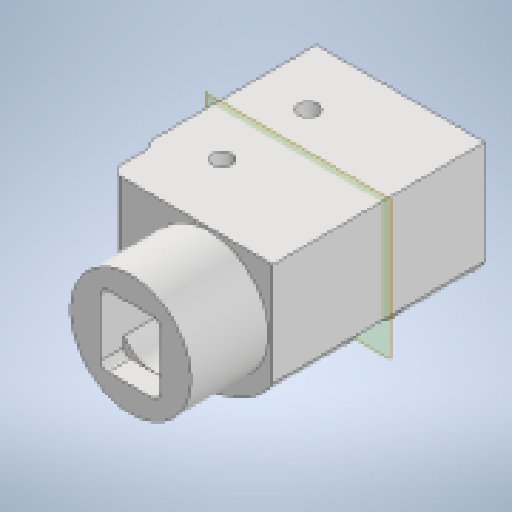
# Autodesk Inventor part: mototrs_Mount_miras_pololu_n20
Saved by Autodesk Inventor 2023.5 (Build 275446000, 446)
## iProperties
Created: 2025-04-06
Part Number: mototrs_Mount_miras_pololu_n20
Material: Ogólny
Document SubType Name: Modeling
Designer: kamil
Density: 1 g/cm^3
Appearance: Domyślna
Author: kamil
Autodesk Inventor part; units mm, degrees
ref_plane "YZ Plane" through (0, 0, 0) normal (1, 0, 0) x (0, 1, 0)
ref_plane "XZ Plane" through (0, 0, 0) normal (0, 1, 0) x (-1, 0, 0)
ref_plane "XY Plane" through (0, 0, 0) normal (0, 0, 1) x (1, 0, 0)
sketch "Szkic1" plane through (0, 0, 0) normal (0, 1, 0) x (-1, 0, 0)
  line L0 (22.5813, 6.7031) -> (-6.8457, 6.7031)
  line L1 (-6.8457, 6.7031) -> (-6.8457, -29.2969)
  line L2 (-6.8457, -29.2969) -> (22.5813, -29.2969)
  line L3 (22.5813, -29.2969) -> (22.5813, 6.7031)
  point P0 (0, 0)
  dimension "d0" = 36
  dimension "d1" = 29.427
  constraints: 8 end point, 2 parallel, 1 horizontal, 1 perpendicular
  measures "d0" distance of L1.end L0.end
  measures "d1" distance of L0.start L0.end
extrude "Wyciągnięcie proste1" add sketch "Szkic1" along normal blind 22
sketch "Szkic2" plane through (-22.5813, 0, 6.7031) normal (0, 0, 1) x (1, 0, 0)
  arc A0 (23.1002, 14.25) -> (13.1002, 14.2503) centre (18.1001, 11.0797) ccw projected
  arc A1 (13.1002, 7.75) -> (23.1002, 7.7503) centre (18.1001, 10.9206) ccw projected
  line L0 (23.1002, 7.7503) -> (23.1002, 14.25)
  line L1 (13.1002, 14.2503) -> (13.1002, 7.75)
  arc A2 (23.2002, 14.2789) -> (13.0002, 14.2792) centre (18.1001, 11.0797) ccw
  line L2 (23.2002, 14.2789) -> (23.2002, 7.7214)
  arc A3 (13.0002, 7.7211) -> (23.2002, 7.7214) centre (18.1001, 10.9206) ccw
  line L3 (13.0002, 7.7211) -> (13.0002, 14.2792)
  point P0 (22.5813, 0)
  dimension "d4" = 0.1
  constraints: 8 end point, 4 point on circle, 2 centre point, 2 parallel, 1 vertical, 3 other
  measures "d4" radial gap between concentric circles of A0 A2
extrude "Wyciągnięcie proste2" cut sketch "Szkic2" against normal blind 5 contours L0 A1 L1 A0 | L2 A3 L3 A2
sketch "Szkic3" plane through (-22.5813, 0, 1.7031) normal (0, 0, 1) x (1, 0, 0)
  line L0 (23.2002, 14.2789) -> (23.2002, 7.7214) projected
  arc A0 (23.2002, 14.2789) -> (13.0002, 14.2792) centre (18.1001, 11.0797) ccw projected
  line L1 (13.0002, 7.7211) -> (13.0002, 14.2792) projected
  arc A1 (13.0002, 7.7211) -> (23.2002, 7.7214) centre (18.1001, 10.9206) ccw projected
  arc A2 (21.7002, 13.8135) -> (14.5002, 13.8137) centre (18.1001, 11.0797) ccw
  line L2 (21.7002, 13.8135) -> (21.7002, 8.1867)
  arc A3 (14.5002, 8.1865) -> (21.7002, 8.1867) centre (18.1001, 10.9206) ccw
  line L3 (14.5002, 8.1865) -> (14.5002, 13.8137)
  point P0 (22.5813, 0)
  dimension "d7" = 1.5
  constraints: 4 end point, 4 point on circle, 2 centre point, 3 other
  measures "d7" distance between parallel lines of L1 L3
extrude "Wyciągnięcie proste3" cut sketch "Szkic3" against normal blind 4 contours L2 A3 L3 A2
ref_plane "Płaszczyzna konstrukcyjna1" through (6.8457, 0, -11.2969) normal (0, 0, -1) x (-1, 0, 0)
sketch "Szkic4" plane through (-22.5813, 0, 6.7031) normal (0, 0, 1) x (1, 0, 0)
  arc A0 (23.2002, 14.2789) -> (13.0002, 14.2792) centre (18.1001, 11.0797) ccw projected
  line L0 (23.2002, 14.2789) -> (23.2002, 7.7214) projected
  arc A1 (13.0002, 7.7211) -> (23.2002, 7.7214) centre (18.1001, 10.9206) ccw projected
  line L1 (13.0002, 7.7211) -> (13.0002, 14.2792) projected
  line L2 (0, 0) -> (29.427, 0) projected
  line L3 (29.427, 0) -> (29.427, 22) projected
  line L4 (0, 22) -> (29.427, 22) projected
  line L5 (0, 0) -> (0, 22) projected
  line L6 (18.1001, 11.0797) -> (18.1001, 10.9206)
  circle A2 centre (18.1001, 11.0001) radius 10.5
  point P0 (22.5813, 0)
  dimension "d10" = 21
  constraints: 2 end point, 1 centre point, 1 coincident, 1 midpoint, 1 vertical
  measures "d10" diameter of A2
extrude "Wyciągnięcie proste4" add sketch "Szkic4" along normal blind 10.5 contours A2
sketch "Szkic5" plane through (-4.4811, 11.0001, 17.2031) normal (0, 0, 1) x (1, 0, 0)
  arc A0 (5.0001, 4.9999) -> (4.0001, 5.9999) centre (4.0001, 4.9999) ccw projected
  line L0 (4.0001, 5.9999) -> (-3.9999, 5.9999) projected
  arc A1 (-3.9999, 5.9999) -> (-4.9999, 4.9999) centre (-3.9999, 4.9999) ccw projected
  line L1 (-4.9999, 4.9999) -> (-4.9999, -5.0001) projected
  arc A2 (-4.9999, -5.0001) -> (-3.9999, -6.0001) centre (-3.9999, -5.0001) ccw projected
  line L2 (-3.9999, -6.0001) -> (4.0001, -6.0001) projected
  arc A3 (4.0001, -6.0001) -> (5.0001, -5.0001) centre (4.0001, -5.0001) ccw projected
  line L3 (5.0001, -5.0001) -> (5.0001, 4.9999) projected
  circle A4 centre (2.7995, -3.8015) radius 1.25 projected
  circle A5 centre (-2.7993, 3.8012) radius 1.25 projected
  circle A6 centre (-1.9632, -3.0148) radius 0.45 projected
  circle A7 centre (1.9634, 3.0145) radius 0.45 projected
  circle A8 centre (0.0001, -4.5001) radius 0.8 projected
  circle A9 centre (0.0001, 4.4999) radius 0.8 projected
  circle A10 centre (0.0001, -0.0001) radius 2 projected
  arc A11 (-3.9999, 6.0999) -> (-5.0999, 4.9999) centre (-3.9999, 4.9999) ccw
  line L4 (-3.9999, 6.0999) -> (4.0001, 6.0999)
  arc A12 (5.1001, 4.9999) -> (4.0001, 6.0999) centre (4.0001, 4.9999) ccw
  line L5 (5.1001, 4.9999) -> (5.1001, -5.0001)
  arc A13 (4.0001, -6.1001) -> (5.1001, -5.0001) centre (4.0001, -5.0001) ccw
  line L6 (4.0001, -6.1001) -> (-3.9999, -6.1001)
  arc A14 (-5.0999, -5.0001) -> (-3.9999, -6.1001) centre (-3.9999, -5.0001) ccw
  line L7 (-5.0999, -5.0001) -> (-5.0999, 4.9999)
  circle A15 centre (0, 0) radius 10.5 projected
  point P0 (4.4811, -11.0001)
  dimension "d13" = 0.1
  constraints: 8 end point, 8 point on circle, 4 centre point, 7 other
  measures "d13" radial gap between concentric circles of A1 A11
ref_plane "Płaszczyzna konstrukcyjna2" through (-9.481, 5, 26.2031) normal (0, 0, 1) x (1, -0.0000003, 0)
ref_plane "Płaszczyzna konstrukcyjna3" through (-9.481, 5, 21.2031) normal (0, 0, 1) x (1, -0.0000003, 0)
extrude "Wyciągnięcie proste5" add sketch "Szkic5" along normal up to surface (4 mm away) contours A15
sketch "Szkic6" plane through (-22.5813, 0, -2.2969) normal (0, 0, 1) x (1, 0, 0)
  line L0 (21.7002, 13.8135) -> (21.7002, 8.1867) projected
  arc A0 (21.7002, 13.8135) -> (14.5002, 13.8137) centre (18.1001, 11.0797) ccw projected
  line L1 (14.5002, 8.1865) -> (14.5002, 13.8137) projected
  arc A1 (14.5002, 8.1865) -> (21.7002, 8.1867) centre (18.1001, 10.9206) ccw projected
  point P0 (22.5813, 0)
extrude "Wyciągnięcie proste6" cut sketch "Szkic6" against normal up to surface (9 mm away)
sketch "Szkic7" plane through (6.8457, 0, 6.7031) normal (1, 0, 0) x (0, 0, -1)
  line L0 (0, 0) -> (36, 0) projected
  line L1 (14, 4) -> (22, 4)
  line L2 (22, 4) -> (22, 0)
  line L3 (22, 0) -> (14, 0)
  line L4 (14, 0) -> (14, 4)
  point P0 (6.7031, 0)
  point P1 (18, 0)
  point P2 (18, 0)
  point P3 (18, 0)
  dimension "d18" = 8
  dimension "d19" = 4
  constraints: 8 end point, 3 midpoint, 2 parallel, 1 coincident, 1 horizontal, 1 horizontal alignment, 1 perpendicular
  measures "d18" distance of L2.end L3.end
  measures "d19" distance of L1.end L2.end
extrude "Wyciągnięcie proste7" cut sketch "Szkic7" against normal through all
sketch "Szkic8" plane through (-8.081, 8.1865, 1.7031) normal (1, 0, 0) x (0, 0, -1)
  line L0 (13, 5.6272) -> (13, 0) projected
  circle A0 centre (13, 2.8136) radius 2.8136
  point P0 (1.7031, -8.1865)
  constraints: 1 midpoint, 3 other
extrude "Wyciągnięcie proste8" cut sketch "Szkic8" against normal through all contours L0 A0 picked at (11.5317, 3.7242)
sketch "Szkic9" plane through (0, 0, 0) normal (0, -1, 0) x (1, 0, 0)
  circle A0 centre (-19.981, -3.7969) radius 1.55 projected
  circle A1 centre (-13.481, -3.7969) radius 1.55 projected
  circle A2 centre (-19.981, -18.7969) radius 1.55 projected
  circle A3 centre (-13.481, -18.7969) radius 1.55 projected
  point P0 (0, 0)
hole "Otwór1" at (-19.981, 0, -18.7969) at (-19.981, 0, -3.7969) direction (0, 1, 0) diameter 3.4 end through all
sketch "Szkic10" plane through (0, 0, 0) normal (0, -1, 0) x (1, 0, 0)
  circle A0 centre (-13.481, -3.7969) radius 1.55 projected
  circle A1 centre (-13.481, -18.7969) radius 1.55 projected
  point P0 (0, 0)
hole "Otwór2" at (-13.481, 0, -18.7969) at (-13.481, 0, -3.7969) direction (0, 1, 0) diameter 3.4 end through all
sketch "Szkic11" plane through (-22.5813, 0, 6.7031) normal (0, 0, 1) x (1, 0, 0)
  circle A0 centre (18.1001, 11.0001) radius 10.5 projected
  line L0 (0, 0) -> (29.427, 0) projected
  line L1 (29.427, 0) -> (29.427, 22) projected
  line L2 (0, 22) -> (29.427, 22) projected
  line L3 (0, 0) -> (0, 22) projected
  point P0 (22.5813, 0)
extrude "Wyciągnięcie proste9" add sketch "Szkic11" along normal blind 1
sketch "Szkic13" plane through (0, 0, 0) normal (0, -1, 0) x (1, 0, 0)
  circle A0 centre (-13.481, -3.7969) radius 1.7 projected
  circle A1 centre (-19.981, -3.7969) radius 1.7 projected
  line L0 (-22.5813, -7.2969) -> (6.8457, -7.2969) projected
  line L1 (6.8457, 7.7031) -> (6.8457, -7.2969) projected
  line L2 (-22.5813, 7.7031) -> (6.8457, 7.7031) projected
  line L3 (-22.5813, -7.2969) -> (-22.5813, 7.7031) projected
  circle A2 centre (-19.981, -3.7969) radius 1.55 projected
  circle A3 centre (-61.7996, -52.0969) radius 1.5 projected
  circle A4 centre (-28.2798, 34.9982) radius 1.6 projected
  circle A5 centre (-61.7996, 29.5031) radius 1.5 projected
  circle A6 centre (-28.2798, -57.5919) radius 1.6 projected
  circle A7 centre (-13.481, -3.7969) radius 1.55 projected
  circle A8 centre (-19.981, -18.7969) radius 1.55 projected
  circle A9 centre (-63.7043, -39.2969) radius 1.6 projected
  circle A10 centre (-29.3543, 16.7031) radius 1.6 projected
  circle A11 centre (-63.7043, 16.7031) radius 1.6 projected
  circle A12 centre (-29.3543, -39.2969) radius 1.6 projected
  circle A13 centre (-13.481, -18.7969) radius 1.55 projected
  arc A14 (-80.181, 31.7031) -> (-81.181, 30.7031) centre (-80.181, 30.7031) ccw projected
  line L4 (-81.181, 30.7031) -> (-81.181, -53.2969) projected
  arc A15 (-81.181, -53.2969) -> (-80.181, -54.2969) centre (-80.181, -53.2969) ccw projected
  line L5 (-80.181, -54.2969) -> (-66.181, -54.2969) projected
  arc A16 (-65.181, -55.2969) -> (-66.181, -54.2969) centre (-66.181, -55.2969) ccw projected
  line L6 (-65.181, -55.2969) -> (-65.181, -60.2969) projected
  arc A17 (-65.181, -60.2969) -> (-64.181, -61.2969) centre (-64.181, -60.2969) ccw projected
  line L7 (-23.181, -61.2969) -> (-64.181, -61.2969) projected
  arc A18 (-23.181, -61.2969) -> (-22.181, -60.2969) centre (-23.181, -60.2969) ccw projected
  line L8 (-22.181, -26.2969) -> (-22.181, -60.2969) projected
  line L9 (-5.181, -26.2969) -> (-22.181, -26.2969) projected
  arc A19 (-5.181, -26.2969) -> (-4.181, -25.2969) centre (-5.181, -25.2969) ccw projected
  line L10 (-4.181, -25.2969) -> (-4.181, 2.7031) projected
  arc A20 (-4.181, 2.7031) -> (-5.181, 3.7031) centre (-5.181, 2.7031) ccw projected
  line L11 (-22.181, 3.7031) -> (-5.181, 3.7031) projected
  line L12 (-22.181, 37.7031) -> (-22.181, 3.7031) projected
  arc A21 (-22.181, 37.7031) -> (-23.181, 38.7031) centre (-23.181, 37.7031) ccw projected
  line L13 (-64.181, 38.7031) -> (-23.181, 38.7031) projected
  arc A22 (-64.181, 38.7031) -> (-65.181, 37.7031) centre (-64.181, 37.7031) ccw projected
  line L14 (-65.181, 37.7031) -> (-65.181, 32.7031) projected
  arc A23 (-66.181, 31.7031) -> (-65.181, 32.7031) centre (-66.181, 32.7031) ccw projected
  line L15 (-66.181, 31.7031) -> (-80.181, 31.7031) projected
  circle A24 centre (-71.5884, -48.5969) radius 3.5 projected
  circle A25 centre (-71.5884, 26.0031) radius 3.5 projected
  circle A26 centre (-13.481, -18.7969) radius 1.7 projected
  circle A27 centre (-19.981, -18.7969) radius 1.7 projected
  line L16 (6.8457, -15.2969) -> (-22.5813, -15.2969) projected
  line L17 (-22.5813, -29.2969) -> (-22.5813, -15.2969) projected
  line L18 (6.8457, -29.2969) -> (-22.5813, -29.2969) projected
  line L19 (6.8457, -15.2969) -> (6.8457, -29.2969) projected
  line L20 (-3.781, 2.7031) -> (-3.781, -25.2969)
  arc A28 (-5.181, -26.6969) -> (-3.781, -25.2969) centre (-5.181, -25.2969) ccw
  line L21 (-5.181, -26.6969) -> (-21.781, -26.6969)
  line L22 (-21.781, -26.6969) -> (-21.781, -60.2969)
  arc A29 (-23.181, -61.6969) -> (-21.781, -60.2969) centre (-23.181, -60.2969) ccw
  line L23 (-23.181, -61.6969) -> (-64.181, -61.6969)
  arc A30 (-65.581, -60.2969) -> (-64.181, -61.6969) centre (-64.181, -60.2969) ccw
  line L24 (-65.581, -60.2969) -> (-65.581, -55.2969)
  arc A31 (-65.581, -55.2969) -> (-66.181, -54.6969) centre (-66.181, -55.2969) ccw
  line L25 (-66.181, -54.6969) -> (-80.181, -54.6969)
  arc A32 (-81.581, -53.2969) -> (-80.181, -54.6969) centre (-80.181, -53.2969) ccw
  line L26 (-81.581, -53.2969) -> (-81.581, 30.7031)
  arc A33 (-80.181, 32.1031) -> (-81.581, 30.7031) centre (-80.181, 30.7031) ccw
  line L27 (-80.181, 32.1031) -> (-66.181, 32.1031)
  arc A34 (-66.181, 32.1031) -> (-65.581, 32.7031) centre (-66.181, 32.7031) ccw
  line L28 (-65.581, 32.7031) -> (-65.581, 37.7031)
  arc A35 (-64.181, 39.1031) -> (-65.581, 37.7031) centre (-64.181, 37.7031) ccw
  line L29 (-64.181, 39.1031) -> (-23.181, 39.1031)
  arc A36 (-21.781, 37.7031) -> (-23.181, 39.1031) centre (-23.181, 37.7031) ccw
  line L30 (-21.781, 37.7031) -> (-21.781, 4.1031)
  line L31 (-21.781, 4.1031) -> (-5.181, 4.1031)
  arc A37 (-3.781, 2.7031) -> (-5.181, 4.1031) centre (-5.181, 2.7031) ccw
  point P0 (0, 0)
  point P1 (-3.781, -15.2969)
  point P2 (-21.781, -29.2969)
  point P3 (-21.781, 7.7031)
  point P4 (-3.781, -7.2969)
  dimension "d42" = 0.4
  constraints: 24 end point, 20 point on circle, 10 centre point, 21 other
  measures "d42" distance between parallel lines of L10 L20
ref_plane "Płaszczyzna konstrukcyjna4" through (-81.181, -3, -61.2969) normal (0, -1, 0) x (1, 0, 0)
extrude "Wyciągnięcie proste11" add sketch "Szkic13" along normal up to surface (3 mm away) contours L20 A37 L31 L30 L2 L1 L0 | L16 L19 L18 L22 L21 A28 L20
sketch "Szkic14" plane through (-22.5813, 0, 7.7031) normal (0, 0, 1) x (1, 0, 0)
  circle A0 centre (18.1001, 11.0001) radius 10.5 projected
  line L0 (0, 0) -> (0.8002, 0) projected
  line L1 (0.8002, 0) -> (0.8002, -3) projected
  line L2 (0.8002, -3) -> (29.427, -3) projected
  line L3 (29.427, 22) -> (29.427, -3) projected
  line L4 (29.427, 22) -> (0, 22) projected
  line L5 (0, 22) -> (0, 0) projected
  circle A1 centre (18.1001, 11.0001) radius 10.5 projected
  circle A2 centre (18.1001, 11.0001) radius 13.3154
  line L6 (19.606, -2.5109) -> (44.0043, 5.4136)
  line L7 (0.8002, -3) -> (29.427, -3) projected
  line L8 (16.5169, -3) -> (0.8002, -3)
  arc A3 (16.5169, -3) -> (19.606, -2.5109) centre (16.5169, 7) ccw
  point P0 (22.5813, 0)
  point P1 (29.427, 4)
  point P2 (18.1001, -3)
  point P3 (22.2134, -1.664)
  dimension "d45" = 10
  constraints: 4 end point, 3 point on line, 2 point on circle, 2 tangent, 1 centre point, 1 coincident, 1 collinear, 1 vertical alignment, 4 other
  measures "d45" radius of A3
extrude "Wyciągnięcie proste12" cut sketch "Szkic14" against normal through all contours A3 L6 L3 L2 | A2 L3 L6
sketch "Szkic15" plane through (0, 22, 0) normal (0, 1, 0) x (1, 0, 0)
  circle A0 centre (-13.481, 18.7969) radius 1.7 projected
  circle A1 centre (-13.481, 3.7969) radius 1.7 projected
  line L0 (6.8457, 29.2969) -> (6.8457, -7.7031) projected
  line L1 (6.8457, 29.2969) -> (-22.5813, 29.2969) projected
  line L2 (-22.5813, 29.2969) -> (-22.5813, -7.7031) projected
  line L3 (6.8457, -7.7031) -> (-22.5813, -7.7031) projected
  arc A2 (-21.481, -5.7031) -> (-19.481, -7.7031) centre (-19.481, -5.7031) ccw projected
  line L4 (-21.481, -5.7031) -> (-21.481, -2.046) projected
  arc A3 (-21.481, -2.046) -> (-22.141, -0.1686) centre (-24.481, -2.046) ccw projected
  arc A4 (-22.581, 1.0829) -> (-22.141, -0.1686) centre (-20.581, 1.0829) ccw projected
  line L5 (-22.581, 1.0829) -> (-22.581, 21.5108) projected
  arc A5 (-22.141, 22.7624) -> (-22.581, 21.5108) centre (-20.581, 21.5108) ccw projected
  line L6 (-21.481, 24.6397) -> (-21.481, 28.2969) projected
  arc A6 (-22.141, 22.7624) -> (-21.481, 24.6397) centre (-24.481, 24.6397) ccw projected
  arc A7 (-19.481, 30.2969) -> (-21.481, 28.2969) centre (-19.481, 28.2969) ccw projected
  line L7 (-30.7464, 11.2969) -> (13.1111, 11.2969) projected
  point P0 (0, 0)
  point P1 (-22.581, 11.2969)
  point P2 (-22.5813, 11.2969)
extrude "Wyciągnięcie proste13" cut sketch "Szkic15" against normal through all contours L3 L2 A4 A3 L4 A2
ref_plane "Płaszczyzna konstrukcyjna5" through (0, 8, 0) normal (0, -1, 0) x (1, 0, 0)
sketch "Szkic16" plane through (0, 8, 0) normal (0, -1, 0) x (1, 0, 0)
  circle A0 centre (-19.981, -3.7969) radius 1.7 projected
  line L0 (-22.581, -11.2969) -> (-22.581, -1.0829) projected
  circle A1 centre (-19.981, -3.7969) radius 2.9
  line L1 (-21.6554, -6.6969) -> (-23.3297, -3.7969)
  line L2 (-23.3297, -3.7969) -> (-21.6554, -0.8969)
  line L3 (-21.6554, -0.8969) -> (-18.3067, -0.8969)
  line L4 (-18.3067, -0.8969) -> (-16.6324, -3.7969)
  line L5 (-16.6324, -3.7969) -> (-18.3067, -6.6969)
  line L6 (-18.3067, -6.6969) -> (-21.6554, -6.6969)
  line L7 (-21.6554, -6.6969) -> (-22.581, -6.6969)
  arc A2 (-22.141, 0.1686) -> (-22.581, -1.0829) centre (-20.581, -1.0829) ccw projected
  arc A3 (-22.141, 0.1686) -> (-22.581, -1.0829) centre (-20.581, -1.0829) ccw projected
  line L8 (-21.6554, -0.8969) -> (-23.6965, -0.8969)
  point P0 (0, 0)
  point P1 (-19.981, -6.6969)
  point P2 (-22.581, -5.0935)
  point P3 (-22.5724, -0.8969)
  point P4 (-22.581, -1.0829)
  point P5 (-22.581, -2.5002)
  dimension "d51" = 5.8
  constraints: 16 end point, 2 coincident, 1 horizontal, 1 midpoint, 1 perpendicular, 1 point on line, 1 vertical alignment, 15 other
extrude "Wyciągnięcie proste14" cut sketch "Szkic16" against normal blind 3
sketch "Szkic17" plane through (0, 22, 0) normal (0, 1, 0) x (1, 0, 0)
  line L0 (-22.5813, 11.2969) -> (-22.581, 11.2969) projected
  line L1 (-22.581, 11.2969) -> (-22.581, 1.0829) projected
  arc A0 (-22.581, 1.0829) -> (-22.141, -0.1686) centre (-20.581, 1.0829) ccw projected
  arc A1 (-21.481, -2.046) -> (-22.141, -0.1686) centre (-24.481, -2.046) ccw projected
  line L2 (-21.481, -2.046) -> (-21.481, -5.7031) projected
  arc A2 (-21.481, -5.7031) -> (-19.481, -7.7031) centre (-19.481, -5.7031) ccw projected
  line L3 (6.8457, -7.7031) -> (-19.481, -7.7031) projected
  line L4 (6.8457, 29.2969) -> (6.8457, -7.7031) projected
  line L5 (6.8457, 29.2969) -> (-22.5813, 29.2969) projected
  line L6 (-22.5813, 29.2969) -> (-22.5813, 11.2969) projected
  circle A3 centre (-19.981, 3.7969) radius 1.7 projected
  circle A4 centre (-19.981, 18.7969) radius 1.7 projected
  circle A5 centre (-13.481, 3.7969) radius 1.7 projected
  circle A6 centre (-13.481, 18.7969) radius 1.7 projected
  line L7 (-30.7464, 11.2969) -> (13.1111, 11.2969) projected
  point P0 (0, 0)
  point P1 (6.8457, 11.2969)
extrude "Wyciągnięcie proste15" cut sketch "Szkic17" against normal through all contours L6 L5 L4 L7
sketch "Szkic18" plane through (6.8457, 4, 7.7031) normal (1, 0, 0) x (0, 0, -1)
  line L0 (19, 0) -> (19, 18) projected
  line L1 (19, 18) -> (0, 18) projected
  line L2 (0, 18) -> (0, 0) projected
  line L3 (0, 0) -> (15, 0) projected
  line L4 (15, 0) -> (19, 0) projected
  line L5 (15, 0) -> (15, -5.664) projected
  line L6 (0, 0) -> (15, 0) projected
  line L7 (0, -5.664) -> (0, 0) projected
  line L8 (0, -5.664) -> (15, -5.664) projected
  point P0 (7.7031, -4)
extrude "Wyciągnięcie proste16" cut sketch "Szkic18" against normal blind 0.327
fillet "Zaokrąglenie2" radius 2 1 edges at (6.5187, 12.7483, 7.7031)
fillet "Zaokrąglenie3" radius 1 3 edges at (5.6419, 13.7882, 7.3579) (5.6422, 8.2131, 7.3577) (-14.9811, 11.0001, 7.7031)
mirror "Odbij1" about plane through (6.8457, 0, -11.2969) normal (0, 0, -1)
sketch "Szkic19" plane through (6.5187, 4, 7.7031) normal (1, 0, 0) x (0, 0, -1)
  line L0 (2, -0.5034) -> (2, 18) projected
  line L1 (15, -0.5034) -> (2, -0.5034) projected
  line L2 (15, 0) -> (15, -0.5034) projected
  line L3 (15, 0) -> (23, 0) projected
  line L4 (23, 0) -> (23, -0.5034) projected
  line L5 (23, -0.5034) -> (36, -0.5034) projected
  line L6 (36, -0.5034) -> (36, 18) projected
  line L7 (36, 18) -> (2, 18) projected
  line L8 (5.2427, 11.4618) -> (10.883, 11.4618) construction
  line L9 (10.883, 11.4618) -> (10.883, 6.9495) construction
  line L10 (10.883, 6.9495) -> (5.2427, 6.9495) construction
  line L11 (5.2427, 6.9495) -> (5.2427, 11.4618) construction
  line L12 (22.6108, 11.4428) -> (30.591, 11.4428) construction
  line L13 (30.591, 11.4428) -> (30.591, 3.2963) construction
  line L14 (30.591, 3.2963) -> (22.6108, 3.2963) construction
  line L15 (22.6108, 3.2963) -> (22.6108, 11.4428) construction
  line L16 (10.0722, 5.3469) -> (6.0435, 5.3469)
  line L17 (6.0435, 5.3469) -> (6.0435, 6.4098)
  line L18 (6.0435, 6.4098) -> (7.3287, 6.4098)
  line L19 (7.3287, 6.4098) -> (7.3287, 9.6377)
  line L20 (7.3287, 9.6377) -> (6.0435, 9.6377)
  line L21 (6.0435, 9.6377) -> (6.0435, 10.6313)
  spline S0 degree 2 poles (6.0435, 10.6313) (6.3252, 10.6313) (6.8838, 10.7055) (7.0519, 10.7845) knots 0 0 0 1 2 2 2
  spline S1 degree 2 poles (7.0519, 10.7845) (7.2447, 10.8834) (7.4622, 11.2146) (7.482, 11.4618) knots 0 0 0 1 2 2 2
  line L22 (7.482, 11.4618) -> (8.8167, 11.4618)
  line L23 (8.8167, 11.4618) -> (8.8167, 6.4098)
  line L24 (8.8167, 6.4098) -> (10.0722, 6.4098)
  line L25 (10.0722, 6.4098) -> (10.0722, 5.3469)
  line L26 (27.4404, 5.328) -> (23.4116, 5.328)
  line L27 (23.4116, 5.328) -> (23.4116, 6.3908)
  line L28 (23.4116, 6.3908) -> (24.6969, 6.3908)
  line L29 (24.6969, 6.3908) -> (24.6969, 9.6188)
  line L30 (24.6969, 9.6188) -> (23.4116, 9.6188)
  line L31 (23.4116, 9.6188) -> (23.4116, 10.6124)
  spline S2 degree 2 poles (23.4116, 10.6124) (23.6934, 10.6124) (24.252, 10.6865) (24.4201, 10.7656) knots 0 0 0 1 2 2 2
  spline S3 degree 2 poles (24.4201, 10.7656) (24.6129, 10.8645) (24.8304, 11.1957) (24.8501, 11.4428) knots 0 0 0 1 2 2 2
  line L32 (24.8501, 11.4428) -> (26.1848, 11.4428)
  line L33 (26.1848, 11.4428) -> (26.1848, 6.3908)
  line L34 (26.1848, 6.3908) -> (27.4404, 6.3908)
  line L35 (27.4404, 6.3908) -> (27.4404, 5.328)
  spline S4 degree 2 poles (32.9176, 7.3943) (32.9176, 6.9148) (32.5913, 6.1041) (32.27, 5.8125) knots 0 0 0 1 2 2 2
  spline S5 degree 2 poles (32.27, 5.8125) (31.9487, 5.5208) (31.0688, 5.1995) (30.4262, 5.1995) knots 0 0 0 1 2 2 2
  spline S6 degree 2 poles (30.4262, 5.1995) (29.744, 5.2044) (28.7652, 5.4269) (28.4439, 5.5702) knots 0 0 0 1 2 2 2
  line L36 (28.4439, 5.5702) -> (28.4439, 6.9)
  line L37 (28.4439, 6.9) -> (28.5823, 6.9)
  spline S7 degree 2 poles (28.5823, 6.9) (28.7009, 6.8357) (28.9877, 6.6676) (29.22, 6.5787) knots 0 0 0 1 2 2 2
  spline S8 degree 2 poles (29.22, 6.5787) (29.4375, 6.4946) (29.8873, 6.3809) (30.1592, 6.3809) knots 0 0 0 1 2 2 2
  spline S9 degree 2 poles (30.1592, 6.3809) (30.3965, 6.3809) (30.9501, 6.4996) (31.1182, 6.6578) knots 0 0 0 1 2 2 2
  spline S10 degree 2 poles (31.1182, 6.6578) (31.2418, 6.7813) (31.3802, 7.0829) (31.3802, 7.335) knots 0 0 0 1 2 2 2
  spline S11 degree 2 poles (31.3802, 7.335) (31.3802, 7.5525) (31.2022, 7.859) (31.0589, 7.9529) knots 0 0 0 1 2 2 2
  spline S12 degree 2 poles (31.0589, 7.9529) (30.8513, 8.0913) (30.2581, 8.1704) (30.0455, 8.1704) knots 0 0 0 1 2 2 2
  spline S13 degree 2 poles (30.0455, 8.1704) (29.7094, 8.1704) (29.0717, 8.0616) (28.8394, 8.0023) knots 0 0 0 1 2 2 2
  line L38 (28.8394, 8.0023) -> (28.7059, 8.0023)
  line L39 (28.7059, 8.0023) -> (28.7059, 11.428)
  line L40 (28.7059, 11.428) -> (32.7495, 11.428)
  line L41 (32.7495, 11.428) -> (32.7495, 10.2762)
  line L42 (32.7495, 10.2762) -> (30.1543, 10.2762)
  line L43 (30.1543, 10.2762) -> (30.1543, 9.2629)
  spline S14 degree 2 poles (30.1543, 9.2629) (30.2779, 9.2727) (30.6189, 9.2826) (30.7129, 9.2826) knots 0 0 0 1 2 2 2
  spline S15 degree 2 poles (30.7129, 9.2826) (31.1528, 9.2826) (31.8943, 9.1047) (32.186, 8.9218) knots 0 0 0 1 2 2 2
  spline S16 degree 2 poles (32.186, 8.9218) (32.532, 8.6944) (32.9176, 7.9381) (32.9176, 7.3943) knots 0 0 0 1 2 2 2
  point P0 (7.7031, -4)
  constraints: 4 other
extrude "Wyciągnięcie proste17" cut sketch "Szkic19" against normal blind 0.4 contours L16 L17 L18 L19 L20 L21 S0 S1 L22 L23 L24 L25 | L26 L27 L28 L29 L30 L31 S2 S3 L32 L33 L34 L35 | S4 S5 S6 L36 L37 S7 S8 S9 S10 S11 S12 S13 L38 L39 L40 L41 L42 L43 S14 S15 S16
sketch "Szkic24" plane through (-4.4811, 11.0001, -43.7969) normal (0, 0, -1) x (-1, 0, 0)
  arc A0 (-4.0001, 6.0999) -> (-5.1001, 4.9999) centre (-4.0001, 4.9999) ccw projected
  line L0 (-4.0001, 6.0999) -> (3.9999, 6.0999) projected
  arc A1 (5.0999, 4.9999) -> (3.9999, 6.0999) centre (3.9999, 4.9999) ccw projected
  line L1 (5.0999, 4.9999) -> (5.0999, -5.0001) projected
  arc A2 (3.9999, -6.1001) -> (5.0999, -5.0001) centre (3.9999, -5.0001) ccw projected
  line L2 (3.9999, -6.1001) -> (-4.0001, -6.1001) projected
  arc A3 (-5.1001, -5.0001) -> (-4.0001, -6.1001) centre (-4.0001, -5.0001) ccw projected
  line L3 (-5.1001, -5.0001) -> (-5.1001, 4.9999) projected
  circle A4 centre (0, 0) radius 10.5 projected
  line L4 (3.9999, 6.1499) -> (-4.0001, 6.1499)
  arc A5 (-4.0001, 6.1499) -> (-5.1501, 4.9999) centre (-4.0001, 4.9999) ccw
  line L5 (-5.1501, 4.9999) -> (-5.1501, -5.0001)
  arc A6 (-5.1501, -5.0001) -> (-4.0001, -6.1501) centre (-4.0001, -5.0001) ccw
  line L6 (-4.0001, -6.1501) -> (3.9999, -6.1501)
  arc A7 (3.9999, -6.1501) -> (5.1499, -5.0001) centre (3.9999, -5.0001) ccw
  line L7 (5.1499, -5.0001) -> (5.1499, 4.9999)
  arc A8 (5.1499, 4.9999) -> (3.9999, 6.1499) centre (3.9999, 4.9999) ccw
  point P0 (-4.4811, -11.0001)
  dimension "d75" = 0.05
  constraints: 8 end point, 8 point on circle, 4 centre point, 7 other
  measures "d75" distance between parallel lines of L0 L4
extrude "Wyciągnięcie proste22" cut sketch "Szkic24" against normal up to surface (4 mm away) contours L0 A1 L1 A2 L2 A3 L3 A0 | A8 L7 A7 L6 A6 L5 A5 L4
sketch "Szkic25" plane through (-0.481, 4.85, -39.7969) normal (0, 0, -1) x (-1, 0, 0)
  line L0 (-1.15, 1.15) -> (-1.15, 11.15) projected
  arc A0 (-1.15, 1.15) -> (0, 0) centre (0, 1.15) ccw projected
  line L1 (8, 0) -> (0, 0) projected
  arc A1 (8, 0) -> (9.15, 1.15) centre (8, 1.15) ccw projected
  line L2 (9.15, 11.15) -> (9.15, 1.15) projected
  arc A2 (9.15, 11.15) -> (8, 12.3) centre (8, 11.15) ccw projected
  line L3 (0, 12.3) -> (8, 12.3) projected
  arc A3 (0, 12.3) -> (-1.15, 11.15) centre (0, 11.15) ccw projected
  line L4 (-1.1, 9.4289) -> (-1.1, 2.8714) projected
  arc A4 (9.1, 9.4292) -> (-1.1, 9.4289) centre (4.0001, 6.2297) ccw projected
  line L5 (9.1, 2.8711) -> (9.1, 9.4292) projected
  arc A5 (-1.1, 2.8714) -> (9.1, 2.8711) centre (4.0001, 6.0706) ccw projected
  line L6 (9.15, 2.8567) -> (9.15, 9.4435)
  arc A6 (9.15, 9.4435) -> (-1.15, 9.4432) centre (4.0001, 6.2297) ccw
  line L7 (-1.15, 9.4432) -> (-1.15, 2.857)
  arc A7 (-1.15, 2.857) -> (9.15, 2.8567) centre (4.0001, 6.0706) ccw
  point P0 (-0.481, -4.85)
  point P1 (9.15, 2.8567)
  point P2 (9.15, 9.4435)
  point P3 (-1.15, 9.4432)
  dimension "d78" = 0.05
  constraints: 4 end point, 4 point on circle, 2 centre point, 3 other
  measures "d78" radial gap between concentric circles of A5 A7
extrude "Wyciągnięcie proste23" cut sketch "Szkic25" against normal up to surface (15.5 mm away) contours L0 A6 L2 A7 | A4 L5 A5 L4
sketch "Szkic26" plane through (6.8457, 0, -11.2969) normal (0, 0, -1) x (-1, 0, 0)
  arc A0 (7.7268, 8.1867) -> (14.9268, 8.1865) centre (11.3269, 10.9206) ccw projected
  arc A1 (14.9268, 13.8137) -> (7.7268, 13.8135) centre (11.3269, 11.0797) ccw projected
  line L0 (11.3269, 10.9206) -> (11.3269, 11.0797)
  arc A2 (14.9268, 13.8137) -> (7.7268, 13.8135) centre (11.3269, 11.0797) ccw projected
  line L1 (7.7268, 13.8135) -> (7.7268, 8.1867) projected
  arc A3 (7.7268, 8.1867) -> (14.9268, 8.1865) centre (11.3269, 10.9206) ccw projected
  line L2 (14.9268, 8.1865) -> (14.9268, 13.8137) projected
  line L3 (6.2268, 14.2789) -> (6.2268, 7.7214) projected
  arc A4 (16.4268, 14.2792) -> (6.2268, 14.2789) centre (11.3269, 11.0797) ccw projected
  line L4 (16.4268, 7.7211) -> (16.4268, 14.2792) projected
  arc A5 (6.2268, 7.7214) -> (16.4268, 7.7211) centre (11.3269, 10.9206) ccw projected
  line L5 (13.8269, 16.5565) -> (8.8269, 16.5565)
  line L6 (8.8269, 16.5565) -> (8.8269, 5.4437)
  line L7 (8.8269, 5.4437) -> (13.8269, 5.4437)
  line L8 (13.8269, 5.4437) -> (13.8269, 16.5565)
  line L9 (13.8269, 16.5565) -> (8.8269, 5.4437) construction
  line L10 (8.8269, 16.5565) -> (13.8269, 5.4437) construction
  point P0 (6.8457, 0)
  point P1 (11.3269, 11.0001)
  point P2 (13.8269, 7.1544)
  point P3 (8.8269, 7.1544)
  point P4 (8.8269, 16.5565)
  point P5 (8.8269, 14.8459)
  point P6 (13.8269, 14.8459)
  dimension "d81" = 5
  constraints: 14 end point, 3 midpoint, 2 parallel, 1 horizontal, 1 perpendicular, 1 point on circle, 1 vertical
  measures "d81" distance of L7.end L6.end
extrude "Wyciągnięcie proste24" cut sketch "Szkic26" along normal mid plane 100 contours A0 L8 L7 L6 | L6 L5 L8 A1 | L7 A5 | A4 L5
